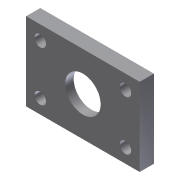
# Autodesk Inventor part: mount pillow block inner bearing capture
Saved by Autodesk Inventor 2012 (Build 160160000, 160)
## iProperties
Created: 2012-04-26
Part Number: mount pillow block inner bearing capture
Material: Default
Document SubType Name: Modeling
Designer: Antonella Wilby
Density: 1 g/cm^3
Author: Antonella Wilby
Autodesk Inventor part; units mm, degrees
ref_plane "YZ Plane" through (0, 0, 0) normal (1, 0, 0) x (0, 1, 0)
ref_plane "XZ Plane" through (0, 0, 0) normal (0, 1, 0) x (-1, 0, 0)
ref_plane "XY Plane" through (0, 0, 0) normal (0, 0, 1) x (1, 0, 0)
sketch "Sketch1" plane through (0, 0, 0) normal (0, 0, 1) x (1, 0, 0)
  circle A0 centre (0, 0) radius 14.2875 construction
  line L0 (-35.56, 0) -> (35.56, 0) projected
  line L1 (0, -24.4475) -> (0, 24.4475) projected
  line L2 (-25.4, 17.4625) -> (25.4, 17.4625)
  line L3 (25.4, 17.4625) -> (25.4, -17.4625)
  line L4 (25.4, -17.4625) -> (-25.4, -17.4625)
  line L5 (-25.4, -17.4625) -> (-25.4, 17.4625)
  circle A1 centre (0, 0) radius 7.9375
  point P0 (0, 17.4625)
  point P1 (-25.4, 0)
  dimension "d0" = 28.575
  dimension "d1" = 50.8
  dimension "d2" = 34.925
  dimension "d3" = 15.875
  constraints: 8 end point, 2 centre point, 2 coincident, 2 midpoint, 2 parallel, 1 horizontal, 1 horizontal alignment, 1 perpendicular, 1 vertical alignment
  measures "d0" diameter of A0
  measures "d1" distance of L2.start L2.end
  measures "d2" distance of L4.end L2.start
  measures "d3" diameter of A1
extrude "Extrusion1" add sketch "Sketch1" along normal mid plane 6.35 contours L5 L2 L1 A1 L0 | L0 A1 L1 L4 L5 | L1 L2 L3 L0 A1 | A1 L0 L3 L4 L1
sketch "Sketch2" plane through (0, 0, -3.175) normal (0, 0, -1) x (-1, 0, 0)
  circle A0 centre (0, 0) radius 7.9375 projected
  circle A1 centre (0, 0) radius 14.3256
  dimension "d6" = 28.6512
  constraints: 1 centre point, 1 coincident
  measures "d6" diameter of A1
extrude "Bearing seat" cut sketch "Sketch2" against normal blind 2.54
sketch "Sketch3" plane through (0, 0, 3.175) normal (0, 0, 1) x (1, 0, 0)
  line L0 (-25.4, 17.4625) -> (25.4, 17.4625) projected
  line L1 (-25.4, -17.4625) -> (-25.4, 17.4625) projected
  line L2 (-35.56, 0) -> (35.56, 0) projected
  line L3 (0, -24.4475) -> (0, 24.4475) projected
  point P0 (-19.05, 11.1125)
  point P1 (19.05, 11.1125)
  point P2 (-19.05, -11.1125)
  point P3 (19.05, -11.1125)
  dimension "d9" = 6.35
  dimension "d10" = 6.35
  constraints: 3 symmetric about line
  measures "d9" distance from line of L0 point (-19.05, 11.112)
  measures "d10" distance from line of L1 point (-19.05, 11.112)
hole "Hole1" at (-19.05, 11.1125, 3.175) at (19.05, 11.1125, 3.175) at (-19.05, -11.1125, 3.175) at (19.05, -11.1125, 3.175) direction (0, 0, -1) diameter 5.1054 end through all clearance for "Flat Head Machine Screw (82)" size "#10" standard "Ansi Unified Screw Threads"
body "Solid1"
